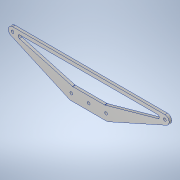
# Autodesk Inventor part: ハンド_上側板
Saved by Autodesk Inventor 2021 (Build 250183000, 183)
## iProperties
Created: 2021-12-06
Part Number: ハンド_上側板
Material: アルミニウム 6061
Document SubType Name: Modeling
Designer: 堀川皓史
Density: 2.7 g/cm^3
Appearance: アルミニウム - フラット
Mass: 41.2556 g
Surface Area: 115.2 cm^2
Volume: 15.2799 cm^3
Author: 堀川皓史
Autodesk Inventor part; units mm, degrees
ref_plane "YZ Plane" through (0, 0, 0) normal (1, 0, 0) x (0, 1, 0)
ref_plane "XZ Plane" through (0, 0, 0) normal (0, 1, 0) x (-1, 0, 0)
ref_plane "XY Plane" through (0, 0, 0) normal (0, 0, 1) x (1, 0, 0)
sketch "スケッチ1" plane through (0, 0, 0) normal (0, 0, 1) x (1, 0, 0)
  circle A0 centre (-20, 0) radius 1.6
  circle A1 centre (20, 0) radius 1.6
  circle A2 centre (0, 0) radius 1.6
  circle A3 centre (-87.5, 27.5) radius 1.6
  circle A4 centre (87.5, 27.5) radius 1.6
  arc A5 (-87.5, 32.5) -> (-89.5442, 22.937) centre (-87.5, 27.5) ccw
  arc A6 (89.5442, 22.937) -> (87.5, 32.5) centre (87.5, 27.5) ccw
  arc A7 (20, -7.5) -> (23.0663, -6.8445) centre (20, 0) ccw
  arc A8 (-23.0663, -6.8445) -> (-20, -7.5) centre (-20, 0) ccw
  line L0 (-89.5442, 22.937) -> (-23.0663, -6.8445)
  line L1 (-87.5, 32.5) -> (87.5, 32.5)
  line L2 (89.5442, 22.937) -> (23.0663, -6.8445)
  line L3 (20, -7.5) -> (-20, -7.5)
  dimension "d0" = 3.2
  dimension "d1" = 3.2
  dimension "d2" = 3.2
  dimension "d3" = 20
  dimension "d4" = 20
  dimension "d5" = 3.2
  dimension "d6" = 3.2
  dimension "d14" = 175
  dimension "d15" = 87.5
  dimension "d17" = 5
  dimension "d18" = 5
  dimension "d19" = 7.5
  dimension "d20" = 7.5
  dimension "d23" = 27.5
  constraints: 9 centre point, 8 end point, 8 point on circle, 8 tangent, 5 coincident, 3 horizontal alignment
  measures "d0" diameter of A0
  measures "d1" diameter of A1
  measures "d2" diameter of A2
  measures "d3" distance of point (0, 0) A0.centre
  measures "d4" distance of point (0, 0) A1.centre
  measures "d5" diameter of A3
  measures "d6" diameter of A4
  measures "d14" distance of A4.centre A3.centre
  measures "d15" horizontal distance of point (0, 0) A3.centre
  measures "d17" radius of A5
  measures "d18" radius of A6
  measures "d19" radius of A8
  measures "d20" radius of A7
  measures "d23" vertical distance of A0.centre A3.centre
extrude "押し出し1" add sketch "スケッチ1" along normal blind 3
sketch "スケッチ2" plane through (0, 0, 3) normal (0, 0, 1) x (1, 0, 0)
  circle A0 centre (-87.5, 27.5) radius 1.6 projected
  arc A1 (-82.937, 25.4558) -> (-82.601, 28.5) centre (-87.5, 27.5) ccw
  circle A2 centre (87.5, 27.5) radius 1.6 projected
  arc A3 (82.601, 28.5) -> (82.937, 25.4558) centre (87.5, 27.5) ccw
  line L0 (-82.601, 28.5) -> (82.601, 28.5)
  line L1 (87.5, 32.5) -> (-87.5, 32.5) projected
  line L2 (-18.3968, 7.5) -> (18.3968, 7.5)
  line L3 (18.3968, 7.5) -> (82.937, 25.4558)
  line L4 (-18.3968, 7.5) -> (-82.937, 25.4558)
  line L5 (-20, -7.5) -> (20, -7.5) projected
  line L6 (-89.5442, 22.937) -> (-23.0663, -6.8445) projected
  line L7 (23.0663, -6.8445) -> (89.5442, 22.937) projected
  point P0 (0, 0)
  dimension "d24" = 5
  dimension "d25" = 5
  dimension "d26" = 4
  dimension "d27" = 15
  dimension "d28" = 15
  dimension "d29" = 15
  dimension "d30" = 5
  dimension "d31" = 5
  constraints: 8 end point, 4 point on circle, 2 centre point, 2 coincident, 1 horizontal, 1 parallel
  measures "d24" radius of A1
  measures "d25" radius of A3
  measures "d26" distance between parallel lines of L1 L0
  measures "d27" distance between parallel lines of L5 L2
  measures "d28" distance from line of L6 L2.start
  measures "d29" distance from line of L7 L2.end
  measures "d30" distance from line of L7 L3.end
  measures "d31" distance from line of L6 L4.end
extrude "押し出し2" cut sketch "スケッチ2" against normal through all contours A1 L0 A3 L3 L2 L4
fillet "フィレット1" radius 2 6 edges at (-82.601, 28.5, 1.5) (-82.937, 25.4558, 1.5) (-18.3968, 7.5, 1.5) (18.3968, 7.5, 1.5) (82.601, 28.5, 1.5) (82.937, 25.4558, 1.5)
equation "\"d15\" = 0.5 * d14"
